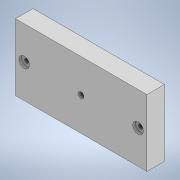
# Autodesk Inventor part: baseblock
Saved by Autodesk Inventor 2022.2 (Build 262287030, 287C)
## iProperties
Created: 2022-02-12
Part Number: baseblock
Material: Generic
Document SubType Name: Modeling
Designer: Tapendra
Density: 1 g/cm^3
Appearance: Default
Author: Tapendra
Autodesk Inventor part; units mm, degrees
ref_plane "YZ Plane" through (0, 0, 0) normal (1, 0, 0) x (0, 1, 0)
ref_plane "XZ Plane" through (0, 0, 0) normal (0, 1, 0) x (-1, 0, 0)
ref_plane "XY Plane" through (0, 0, 0) normal (0, 0, 1) x (1, 0, 0)
sketch "Sketch1" plane through (0, 0, 0) normal (0, 0, 1) x (1, 0, 0)
  line L0 (-37.5, 19) -> (37.5, 19)
  line L1 (37.5, 19) -> (37.5, -19)
  line L2 (37.5, -19) -> (-37.5, -19)
  line L3 (-37.5, -19) -> (-37.5, 19)
  line L4 (-37.5, 19) -> (37.5, -19) construction
  line L5 (37.5, 19) -> (-37.5, -19) construction
  point P0 (0, 0)
  dimension "d2" = 38
  dimension "d3" = 75
  constraints: 12 end point, 2 midpoint, 2 parallel, 1 horizontal, 1 perpendicular
  measures "d2" distance between parallel lines of L0 L2
  measures "d3" distance between parallel lines of L3 L1
extrude "Extrusion1" add sketch "Sketch1" along normal mid plane 10
sketch "Sketch3" plane through (0, 0, 5) normal (0, 0, 1) x (1, 0, 0)
  point P0 (0, 0)
  point P1 (0, 0)
  constraints: 1 coincident
hole "Hole2" at (0, 0, 5) direction (0, 0, -1) diameter 3.175 depth 5 tip angle 118
sketch "Sketch4" plane through (0, 0, 5) normal (0, 0, 1) x (1, 0, 0)
  line L0 (-37.5, 19) -> (-37.5, -19) projected
  circle A0 centre (0, 0) radius 1.5875 projected
  line L1 (-37.5, -19) -> (37.5, -19) projected
  line L2 (37.5, -19) -> (37.5, 19) projected
  line L3 (37.5, 19) -> (-37.5, 19) projected
  line L4 (-37.5, 19) -> (-37.5, -19) projected
  point P0 (-32.5, 0)
  point P1 (32.5, 0)
  dimension "d76" = 5
  dimension "d79" = 65
  constraints: 1 horizontal, 1 other
  measures "d76" distance from line of L0 point (-32.5, 0)
  measures "d79" distance of point (-32.5, 0) point (32.5, 0)
hole "Hole3" at (-32.5, 0, 5) at (32.5, 0, 5) direction (0, 0, -1) diameter 2.459 end through all counterbore diameter 6 counterbore depth 1.4 thread size "M3x0.5" class "6H" standard "ANSI Metric M Profile"
body "Solid1"
